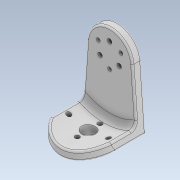
# Autodesk Inventor part: shank_thigh_connector
Saved by Autodesk Inventor 2020 (Build 240168000, 168)
## iProperties
Created: 2021-01-06
Part Number: shank_thigh_connector
Material: Generic
Document SubType Name: Modeling
Designer: DELL
Density: 1 g/cm^3
Appearance: Clear - Blue
Author: DELL
Autodesk Inventor part; units mm, degrees
ref_plane "YZ Plane" through (0, 0, 0) normal (1, 0, 0) x (0, 1, 0)
ref_plane "XZ Plane" through (0, 0, 0) normal (0, 1, 0) x (-1, 0, 0)
ref_plane "XY Plane" through (0, 0, 0) normal (0, 0, 1) x (1, 0, 0)
sketch "Sketch1" plane through (0, 0, 0) normal (0, 0, 1) x (1, 0, 0)
  circle A0 centre (0, 0) radius 20
  line L0 (-19.9445, 1.4891) -> (-23.9583, -52.2709)
  line L1 (19.9445, 1.4891) -> (23.9583, -52.2709)
  line L2 (9.9593, -5.75) -> (0, 0) construction
  circle A1 centre (8.4134, -4.8575) radius 2
  line L3 (0, 0) -> (9.9593, 5.75) construction
  line L4 (0, 0) -> (-9.9593, -5.75) construction
  circle A2 centre (-8.4134, -4.8575) radius 2
  circle A3 centre (0, 0) radius 9.715 construction
  circle A4 centre (0, 0) radius 11.5 construction
  circle A5 centre (0, 9.715) radius 2
  line L5 (0, 0) -> (-9.9593, 5.75) construction
  line L6 (11.5, 0) -> (-11.5, 0) construction
  circle A6 centre (-9.9593, 5.75) radius 2.75
  circle A7 centre (-9.9593, 5.75) radius 1.65
  line L7 (0, -48.5721) -> (0, 22.5) construction
  circle A8 centre (0, -11.5) radius 1.65
  circle A9 centre (0, -11.5) radius 2.75
  circle A10 centre (9.9593, 5.75) radius 2.75
  circle A11 centre (9.9593, 5.75) radius 1.65
  arc A12 (-23.3564, -44.2095) -> (23.3564, -44.2095) centre (0, 0) ccw
  arc A13 (-23.9583, -52.2709) -> (23.9583, -52.2709) centre (0, 0) ccw
  line L8 (0, 0) -> (-23.9583, -52.2709) construction
  point P0 (0, 11.4686)
  point P1 (0, 11.4686)
  point P2 (11.5, 0)
  point P3 (-11.5, 0)
  dimension "d18" = 23
  dimension "d0" = 40
  dimension "d17" = 19.43
  dimension "d19" = 30
  dimension "d20" = 30
  dimension "d21" = 3.3
  dimension "d22" = 5.5
  dimension "d23" = 4
  dimension "d24" = 100
  dimension "d25" = 115
  dimension "d58" = 24.624
  constraints: 16 end point, 13 centre point, 10 coincident, 9 point on circle, 8 point on line, 6 equal radius, 2 tangent, 1 vertical, 17 other
  measures "d0" diameter of A0
  measures "d17" diameter of A3
  measures "d19" angle to the sketch x axis of L5
  measures "d20" angle to the sketch x axis of L4
  measures "d21" diameter of A11
  measures "d22" diameter of A10
  measures "d23" diameter of A5
  measures "d24" diameter of A12
  measures "d25" diameter of A13
  measures "d58" angle of L7 L8
extrude "Extrusion1" add sketch "Sketch1" along normal blind 8 contours A0 | A0 L1 A12 L0 | L1 A13 L0 A12 | A1 | A2 | A5 | A6 | A9 | A10
extrude "Extrusion2" cut sketch "Sketch1" along normal blind 5 contours A6 | A9 | A10 | A11
extrude "Extrusion3" cut sketch "Sketch1" against normal blind 5 from surface at 8 contours A1 | A2 | A5
extrude "Extrusion4" add sketch "Sketch1" along normal blind 45 from surface at 8 contours L1 A13 L0 A12
sketch "Sketch3" plane through (0, 0, 0) normal (0, 1, 0) x (-1, 0, 0)
  circle A0 centre (1.0417, 15.5) radius 2
  circle A1 centre (1.0417, 35.5) radius 2
  circle A2 centre (1.0417, 35.5) radius 1.25
  circle A3 centre (1.0417, 15.5) radius 1.25
  line L0 (-23.9583, 25.5) -> (24.0351, 25.5) construction
  line L1 (1.0417, 9.7156) -> (1.0417, 41.2844) construction
  circle A4 centre (-16.4583, 25.5) radius 1.25
  circle A5 centre (-16.4583, 25.5) radius 2
  circle A6 centre (18.5417, 25.5) radius 1.25
  circle A7 centre (18.5417, 25.5) radius 2
  circle A8 centre (1.0417, 25.5) radius 6
  circle A9 centre (1.0417, 25.5) radius 25
  line L2 (23.3564, 53) -> (-23.3564, 53) projected
  line L3 (23.9583, 35.4913) -> (23.9583, 53)
  line L4 (23.9583, 53) -> (-23.9583, 53)
  line L5 (-23.9583, 53) -> (-23.9583, 25.5)
  line L6 (23.9583, 0) -> (23.9583, 53) projected
  line L7 (-23.9583, 0) -> (-23.9583, 53) projected
  point P0 (0, 0)
  point P1 (-23.9583, 25.5)
  dimension "d47" = 50
  dimension "d42" = 4
  dimension "d43" = 2.5
  dimension "d44" = 20
  dimension "d45" = 35
  dimension "d46" = 12
  dimension "d60" = 27.5
  constraints: 10 end point, 9 centre point, 6 equal radius, 5 coincident, 4 point on line, 3 collinear, 2 perpendicular, 2 symmetric about line, 2 vertical, 1 horizontal, 1 midpoint, 3 other
  measures "d42" diameter of A1
  measures "d43" diameter of A2
  measures "d44" distance of A1.centre A0.centre
  measures "d45" distance of A6.centre A4.centre
  measures "d46" diameter of A8
  measures "d60" distance between parallel lines of L2 L0
extrude "Extrusion8" cut sketch "Sketch3" against normal through all contours A2 | A3 | A4 | A6 | A8 | A9 L5 L4 L2 L3
extrude "Extrusion13" cut sketch "Sketch3" against normal blind 53 contours A0 | A1 | A2 | A3 | A4 | A5 | A6 | A7
fillet "Fillet1" radius 5 1 edges at (0, -50, 8)
fillet "Fillet2" radius 1.5 15 edges at (0, -57.5, 0) (23.9583, -52.2709, 12.75) (-23.9583, -52.2709, 17.7457) (-21.9514, -25.3909, 0) (21.9514, -25.3909, 0) (0, 20, 0) (-21.4452, -18.6106, 8) (-23.2297, -42.5117, 9.3756) (-23.3564, -44.2095, 24.8858) (21.4452, -18.6106, 8) (23.2297, -42.5117, 9.3756) (23.3564, -44.2095, 21.9764) (0, 20, 8) (3.0655, -49.9059, 50.1603) (5.84, -57.2027, 49.5342)
body "Solid1"
